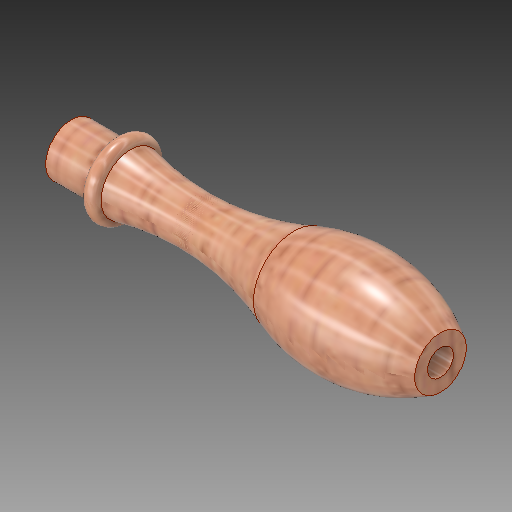
# Autodesk Inventor part: Mango
Saved by Autodesk Inventor 2020 (Build 240168000, 168)
## iProperties
Created: 2016-05-05
Part Number: Mango
Material: Wood (Oak)
Document SubType Name: Modeling
Designer: Jorge
Mass: 9.84021 g
Surface Area: 54.2145 cm^2
Volume: 12.9476 cm^3
Density: 0.76 g/cm^3
Appearance: White Oak - Natural Medium Gloss
Author: Jorge
Autodesk Inventor part; units mm, degrees
ref_plane "YZ Plane" through (0, 0, 0) normal (1, 0, 0) x (0, 1, 0)
ref_plane "XZ Plane" through (0, 0, 0) normal (0, 1, 0) x (-1, 0, 0)
ref_plane "XY Plane" through (0, 0, 0) normal (0, 0, 1) x (1, 0, 0)
sketch "Sketch1" plane through (0, 0, 0) normal (0, 0, 1) x (1, 0, 0)
  line L0 (-15.952, 0) -> (95.7118, 0) projected
  line L1 (0, -41.4801) -> (0, 82.1932) construction
  line L2 (0, 5.5563) -> (9.525, 5.5563)
  arc A0 (12.7, 6.35) -> (9.525, 6.35) centre (11.1125, 6.35) ccw
  line L3 (9.525, 5.5563) -> (9.525, 6.35)
  line L4 (49.0333, 11.1125) -> (60.4744, 11.1125) construction
  line L5 (25.177, 4.7625) -> (44.7051, 4.7625) construction
  line L6 (6.9095, 7.9375) -> (19.8278, 7.9375) construction
  line L7 (11.1125, 6.35) -> (14.4696, 6.35) construction
  arc A1 (12.7, 6.35) -> (47.9001, 8.7704) centre (26.3831, 64.5256) ccw
  arc A2 (79.375, 5.5563) -> (47.9001, 8.7704) centre (60.4744, -23.8125) ccw
  line L8 (12.7, 9.8172) -> (12.7, 3.2434) construction
  line L9 (0, 2.7781) -> (0, 5.5563)
  line L10 (79.375, 5.5563) -> (79.375, 2.7781)
  line L11 (0, 2.7781) -> (79.375, 2.7781)
  point P0 (0, 0)
  point P1 (26.9875, 4.7625)
  point P2 (60.325, 11.1125)
  dimension "d3" = 11.1125
  dimension "d5" = 0
  dimension "d8" = 9.525
  dimension "d10" = 26.9875
  dimension "d13" = 60.325
  dimension "d14" = 22.225
  dimension "d16" = 9.525
  dimension "d20" = 15.875
  dimension "d21" = 59.7631
  dimension "d22" = 34.925
  dimension "d25" = 3.175
  dimension "d27" = 79.375
  dimension "d28" = 11.1125
  dimension "d29" = 5.5563
  constraints: 20 end point, 7 point on circle, 6 horizontal, 6 tangent, 4 point on line, 3 centre point, 3 vertical
  measures "d3" diameter of L2 L0
  measures "d5" distance from line of L1 L2.start
  measures "d8" distance from line of L1 L2.end
  measures "d10" distance from line of point (26.988, 4.763) L1
  measures "d13" distance from line of L1 point (60.325, 11.113)
  measures "d14" diameter of point (60.325, 11.113) L0
  measures "d16" diameter of point (26.988, 4.763) L0
  measures "d20" diameter of L6 L0
  measures "d21" radius of A1
  measures "d22" radius of A2
  measures "d25" distance between parallel lines of L8 L3
  measures "d27" distance from line of L10.start L1
  measures "d28" diameter of L10.start L0
  measures "d29" diameter of L11 L0
revolve "Revolution1" add sketch "Sketch1" angle 360 about axis through (-10, 0, 0) along (1, 0, 0)
body "Solid1"
